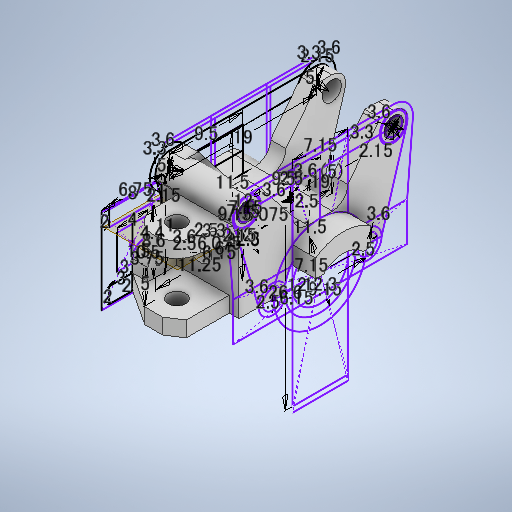
# Autodesk Inventor part: ikafly6.0_2.5d
Saved by Autodesk Inventor 2025 (Build 290162000, 162)
## iProperties
Created: 2024-06-20
Part Number: ikafly6.0_2.5d
Material: 一般
Document SubType Name: Modeling
Designer: Saigusa
Density: 1 g/cm^3
Appearance: 既定
Author: Saigusa
Autodesk Inventor part; units mm, degrees
ref_plane "YZ Plane" through (0, 0, 0) normal (1, 0, 0) x (0, 1, 0)
ref_plane "XZ Plane" through (0, 0, 0) normal (0, 1, 0) x (-1, 0, 0)
ref_plane "XY Plane" through (0, 0, 0) normal (0, 0, 1) x (1, 0, 0)
sketch "スケッチ1" plane through (0, 0, 0) normal (1, 0, 0) x (0, 1, 0)
  circle A0 centre (0, 0) radius 4.575
  circle A1 centre (0, 0) radius 3.575
  line L0 (0, 0) -> (0, 6)
  line L1 (0, 6) -> (0, -6)
  line L2 (0, 0) -> (11.5, 0)
  line L3 (11.5, 0) -> (11.5, 9.5)
  line L4 (11.5, 9.5) -> (11.5, -9.5)
  circle A2 centre (11.5, 9.5) radius 1.65
  circle A3 centre (11.5, -9.5) radius 1.65
  line L5 (0, 0) -> (0, 11.25)
  line L6 (0, 11.25) -> (0, -11.25)
  line L7 (-2.5, -11.25) -> (2.5, -11.25)
  line L8 (2.5, -11.25) -> (2.5, 11.25)
  line L9 (2.5, 11.25) -> (-2.5, 11.25)
  line L10 (-2.5, 11.25) -> (-2.5, -11.25)
  line L11 (-2.5, -11.25) -> (2.5, 11.25) construction
  line L12 (2.5, -11.25) -> (-2.5, 11.25) construction
  circle A4 centre (11.5, 9.5) radius 2.5
  circle A5 centre (11.5, -9.5) radius 2.5
  line L13 (2.5, 11.25) -> (11.2899, 11.9912)
  line L14 (2.5, -11.25) -> (11.2899, -11.9912)
  line L15 (14, 9.5) -> (14, -9.5)
  line L16 (0, -3.575) -> (14, -3.575)
  line L17 (0, 3.575) -> (14, 3.575)
  circle A6 centre (0, 0) radius 6
  line L18 (0, 0) -> (0, 6.15)
  line L19 (0, 6.15) -> (0, -6.15)
  circle A7 centre (0, 6.15) radius 1.25
  circle A8 centre (0, -6.15) radius 1.25
  line L20 (0, 0) -> (0, -6.075)
  line L21 (0, 0) -> (0, 6.075)
  circle A9 centre (0, -6.075) radius 1.25
  circle A10 centre (0, 6.075) radius 1.25
  circle A11 centre (11.5, 9.5) radius 1.075
  circle A12 centre (11.5, -9.5) radius 1.075
  circle A13 centre (11.5, -9.5) radius 1.8
  circle A14 centre (11.5, 9.5) radius 1.8
  line L22 (11.5, -9.5) -> (13.3, -9.5)
  line L23 (11.5, 9.5) -> (13.3, 9.5)
  line L24 (13.3, -9.5) -> (13.3, 9.5)
  circle A15 centre (0, -6.15) radius 1.8
  circle A16 centre (0, 6.15) radius 1.8
  line L25 (0, -7.95) -> (10.9858, -11.225)
  line L26 (0, 7.95) -> (10.9858, 11.225)
  line L27 (0, 11.3) -> (0, 0)
  line L28 (0, 0) -> (11.5, 0)
  line L29 (11.5, 0) -> (11.5, 11.3)
  line L30 (0, 0) -> (8.6, 0)
  line L31 (8.6, 0) -> (8.6, 10.5138)
  line L32 (8.6, 10.5138) -> (0, 10.5138)
  line L33 (0, 10.5138) -> (0, 0)
  line L34 (0, 10.5138) -> (2, 10.5138)
  line L35 (2, 10.5138) -> (2, 14.2638)
  line L36 (2, 14.2638) -> (0, 14.2638)
  line L37 (0, 14.2638) -> (0, 10.5138)
  line L38 (0, 14.2638) -> (2, 14.2638)
  line L39 (2, 14.2638) -> (2, 17.2638)
  line L40 (2, 17.2638) -> (0, 17.2638)
  line L41 (0, 17.2638) -> (0, 14.2638)
  line L42 (0, 10.5138) -> (8.6, 10.5138)
  line L43 (8.6, 10.5138) -> (8.6, 14.2638)
  line L44 (8.6, 14.2638) -> (0, 14.2638)
  line L45 (0, 14.2638) -> (0, 10.5138)
  line L46 (8.6, 10.5138) -> (10.6, 10.5138)
  line L47 (10.6, 10.5138) -> (10.6, 17.2638)
  line L48 (10.6, 17.2638) -> (8.6, 17.2638)
  line L49 (8.6, 17.2638) -> (8.6, 10.5138)
  line L50 (3.1, 16.2638) -> (7.5, 16.2638)
  line L51 (7.5, 16.2638) -> (7.5, 12.2638)
  line L52 (7.5, 12.2638) -> (3.1, 12.2638)
  line L53 (3.1, 12.2638) -> (3.1, 16.2638)
  line L54 (3.1, 16.2638) -> (7.5, 12.2638) construction
  line L55 (7.5, 16.2638) -> (3.1, 12.2638) construction
  line L56 (3.1, 14.2638) -> (3.6, 14.2638)
  line L57 (3.6, 14.2638) -> (3.6, 12.7638)
  line L58 (3.6, 12.7638) -> (3.1, 12.7638)
  line L59 (3.1, 12.7638) -> (3.1, 14.2638)
  circle A17 centre (3.6, 12.7638) radius 0.5
  circle A18 centre (3.6, 12.7638) radius 1.5
  line L60 (3.6, 12.7638) -> (5.1, 12.7638)
  line L61 (5.1, 12.7638) -> (5.1, 10.5138)
  line L62 (5.1, 10.5138) -> (3.6, 10.5138)
  line L63 (3.6, 10.5138) -> (3.6, 12.7638)
  line L64 (11.5, 7.7) -> (0, 7.7)
  line L65 (10.6, 10.5138) -> (11.1423, 10.5138)
  line L66 (0, 7.7) -> (10.6, 7.7)
  line L67 (10.6, 7.7) -> (10.6, 10.5138)
  line L68 (10.6, 10.5138) -> (0, 10.5138)
  line L69 (0, 10.5138) -> (0, 7.7)
  line L70 (-0.2, 18.2638) -> (10.8, 18.2638)
  line L71 (10.8, 18.2638) -> (10.8, 10.2638)
  line L72 (10.8, 10.2638) -> (-0.2, 10.2638)
  line L73 (-0.2, 10.2638) -> (-0.2, 18.2638)
  line L74 (-0.2, 18.2638) -> (10.8, 10.2638) construction
  line L75 (10.8, 18.2638) -> (-0.2, 10.2638) construction
  point P0 (0, 4.575)
  point P1 (0, -4.575)
  point P2 (2.5, 3.575)
  point P3 (2.5, 2.5555)
  point P4 (2.5, -2.5555)
  point P5 (2.5, -3.575)
  point P6 (0, 7.4)
  point P7 (0, 4.9)
  point P8 (0, -4.9)
  point P9 (0, -7.4)
  point P10 (2.5, 5.4544)
  point P11 (2.5, -5.4544)
  point P12 (4.8186, 3.575)
  point P13 (4.8186, -3.575)
  point P14 (2.8548, 3.575)
  point P15 (2.8548, -3.575)
  point P16 (0, 7.95)
  point P17 (2.5, -8.6953)
  point P18 (2.5, 8.6953)
  point P19 (5.3, 14.2638)
  point P20 (3.2258, 11.3112)
  point P21 (3.6, 11.3428)
  point P22 (3.6, 11.2638)
  point P23 (11.5, 7.85)
  point P24 (10.1982, 10.5138)
  point P25 (10.6, 8.1171)
  point P26 (11.5, 8.425)
  point P27 (11.5, 10.575)
  point P28 (10.0126, 10.5138)
  point P29 (10.6, 11.933)
  point P30 (8.6, 11.7643)
  point P31 (10.7435, 10.2638)
  point P32 (10.8, 10.3159)
  point P33 (10.8, 11.1696)
  point P34 (10.6, 11.11)
  point P35 (8.6, 10.2638)
  point P36 (10.8, 10.5138)
  dimension "d110" = 2.15
  dimension "d114" = 3.6
  dimension "d115" = 3.6
  dimension "d0" = 9.15
  dimension "d1" = 7.15
  dimension "d2" = 6
  dimension "d3" = 12
  dimension "d6" = 11.5
  dimension "d7" = 9.5
  dimension "d8" = 19
  dimension "d9" = 3.3
  dimension "d10" = 3.3
  dimension "d11" = 11.25
  dimension "d12" = 22.5
  dimension "d13" = 5
  dimension "d14" = 5
  dimension "d15" = 5
  dimension "d28" = 12
  dimension "d29" = 6.15
  dimension "d30" = 12.3
  dimension "d31" = 2.5
  dimension "d32" = 2.5
  dimension "d99" = 6.075
  dimension "d100" = 6.075
  dimension "d101" = 2.5
  dimension "d102" = 2.5
  dimension "d111" = 2.15
  dimension "d112" = 3.6
  dimension "d113" = 3.6
  dimension "d133" = 8.6
  dimension "d134" = 2
  dimension "d135" = 3.75
  dimension "d136" = 2
  dimension "d137" = 3
  dimension "d138" = 2
  dimension "d139" = 6.75
  dimension "d140" = 4.4
  dimension "d141" = 4
  dimension "d142" = 0.5
  dimension "d143" = 1.5
  dimension "d144" = 3
  dimension "d174" = 11
  dimension "d175" = 8
  constraints: 152 end point, 25 parallel, 19 coincident, 18 point on line, 15 centre point, 15 perpendicular, 13 horizontal, 12 point on circle, 8 tangent, 7 midpoint, 2 vertical alignment, 1 horizontal alignment, 1 vertical, 9 other
  measures "d0" diameter of A0
  measures "d1" diameter of A1
  measures "d2" distance of L0.start L0.end
  measures "d3" distance of L0.end L1.end
  measures "d6" distance of L0.start L2.end
  measures "d7" distance of L2.end L3.end
  measures "d8" distance of L3.end L4.end
  measures "d9" diameter of A2
  measures "d10" diameter of A3
  measures "d11" distance of L0.start L5.end
  measures "d12" distance of L5.end L6.end
  measures "d13" distance of L9.end L8.end
  measures "d14" diameter of A4
  measures "d15" diameter of A5
  measures "d28" diameter of A6
  measures "d29" distance of L18.start L18.end
  measures "d30" distance of L18.end L19.end
  measures "d31" diameter of A7
  measures "d32" diameter of A8
  measures "d99" distance of L18.start L20.end
  measures "d100" distance of L18.start L21.end
  measures "d101" diameter of A9
  measures "d102" diameter of A10
  measures "d111" diameter of A12
  measures "d112" diameter of A13
  measures "d113" diameter of A14
  measures "d133" distance of L32.end L31.end
  measures "d134" distance of L36.end L35.end
  measures "d135" distance of L35.end L34.end
  measures "d136" distance of L40.end L39.end
  measures "d137" distance of L39.end L38.end
  measures "d138" distance of L48.end L47.end
  measures "d139" distance of L47.end L46.end
  measures "d140" distance of L51.end L52.end
  measures "d141" distance of L50.end L51.end
  measures "d142" distance of L57.end L58.end
  measures "d143" distance of L56.end L57.end
  measures "d144" diameter of A18
  measures "d174" distance of L71.end L72.end
  measures "d175" distance of L70.end L71.end
extrude "押し出し7" add sketch "スケッチ1" along normal blind 2 contours L2 A6 L16 A0 | A0 L17 A6 L2 | A0 L8 A6 L17 | L16 A6 L8 A0 | A6 L17 L31 L2 | L2 L4 L16 A6 | A0 A16 A6 L8 | A6 L8 L64 L31 L17 | L8 A6 A15 A0 | L16 L4 A5 L25 L8 A6 | L31 L17 L3 L2 | A0 L0 A10 A6 A16 | A6 A16 L64 L8 | L31 L64 A4 L3 L17 | A15 A6 A9 L1 A0 | L8 L25 A15 A6 | L16 L24 A5 L4 | L4 L3 L17 L24 L16 | A6 A10 L5 L64 A16 | L64 A16 L26 L8 | L8 L26 L72 L31 L64 | L3 A4 L24 L17 | L31 L72 A4 L64 | A15 L6 A8 A6 | A5 L24 A13 L4 | L4 A13 L25 A5 | L0 A7 A6 A10 | L64 L5 A16 | A4 L64 L3 | L3 A14 L24 A4 | L72 L26 L31 | L31 L46 A4 L72 | A4 L72 A14 L67 L64 | A9 A6 A8 L1 | A13 L22 A3 L4 | L4 A3 L22 A13 | A14 L67 A2 L3 | L3 A2 L23 A14 | L64 L67 A14 | L26 A4 L46 | A4 L46 A14 L72 | L23 A2 L29 A14 | A14 L72 A2 L67 | L26 L47 A14 L46 A4 | A14 L46 A2 L72 | L29 A2 L71 A14 | L26 L71 A14 L47 | A14 L47 A2 L46 | A14 L71 L26 | A14 L71 A2 L47 picked at (1.3383, 5.2331) picked at (1.3383, -5.2331) picked at (0.0969, 4.8614) picked at (0.0969, -4.8614)
extrude "押し出し8" add sketch "スケッチ1" along normal blind 10 contours L2 A6 L16 A0 | A0 L17 A6 L2 | A0 L8 A6 L17 | L16 A6 L8 A0 | A6 L17 L31 L2 | L2 L4 L16 A6 | A0 A16 A6 L8 | L8 A6 A15 A0 | L31 L17 L3 L2 | A0 L0 A10 A6 A16 | A6 A16 L64 L8 | A15 A6 A9 L1 A0 | L8 L25 A15 A6 | L4 L3 L17 L24 L16 | A6 A10 L5 L64 A16 | L64 A16 L26 L8 | A15 L6 A8 A6 | L24 L17 L15 L16 | L0 A7 A6 A10 | A6 L5 A10 | L64 L5 A16 | A9 A6 A8 L1 | L0 A6 A7 | A8 A6 L1 | A8 L6 A6 picked at (1.3383, 5.2331) picked at (1.3383, -5.2331) picked at (0.0969, 4.8614) picked at (0.0969, -4.8614) picked at (0.2292, 5.6392) picked at (0.2292, -5.6392)
sketch "スケッチ6" plane through (10, 0, 0) normal (1, 0, 0) x (0, 0, -1)
  line L0 (0, 0) -> (-6.15, 0)
  line L1 (-6.15, 0) -> (6.15, 0)
  circle A0 centre (-6.15, 0) radius 1.25
  circle A1 centre (6.15, 0) radius 1.25
  line L2 (-11.25, 2.5) -> (11.25, 2.5)
  line L3 (11.25, 2.5) -> (11.25, -2.5)
  line L4 (11.25, -2.5) -> (-11.25, -2.5)
  line L5 (-11.25, -2.5) -> (-11.25, 2.5)
  line L6 (-11.25, 2.5) -> (11.25, -2.5) construction
  line L7 (11.25, 2.5) -> (-11.25, -2.5) construction
  line L8 (0, 0) -> (0, 11.5)
  line L9 (0, 11.5) -> (-9.5, 11.5)
  line L10 (-9.5, 11.5) -> (9.5, 11.5)
  circle A2 centre (-9.5, 11.5) radius 1.65
  circle A3 centre (9.5, 11.5) radius 1.65
  circle A4 centre (0, 0) radius 6
  circle A5 centre (0, 0) radius 4.575
  arc A6 (11.9912, 11.2899) -> (9.5, 14) centre (9.5, 11.5) ccw
  line L11 (11.25, 2.5) -> (11.9912, 11.2899)
  line L12 (-11.25, 2.5) -> (-11.9912, 11.2899)
  line L13 (-9.5, 14) -> (9.5, 14)
  circle A7 centre (0, 0) radius 3.575
  line L14 (-3.575, 14) -> (-3.575, 4.8186)
  line L15 (3.575, -14) -> (-3.575, -14)
  line L16 (-3.575, 14) -> (3.575, 14)
  line L17 (3.575, 14) -> (3.575, -14)
  line L18 (3.575, -14) -> (-3.575, 14) construction
  line L19 (-3.575, -14) -> (3.575, 14) construction
  circle A8 centre (-9.5, 11.5) radius 1.075
  circle A9 centre (9.5, 11.5) radius 1.075
  circle A10 centre (9.5, 11.5) radius 1.8
  circle A11 centre (-9.5, 11.5) radius 1.8
  line L20 (-9.5, 11.5) -> (-9.5, 13.3)
  line L21 (-9.5, 13.3) -> (9.5, 13.3)
  circle A12 centre (-6.15, 0) radius 1.8
  circle A13 centre (6.15, 0) radius 1.8
  line L22 (-7.95, 0) -> (-11.225, 10.9858)
  line L23 (4.575, 0) -> (7.95, 0)
  line L24 (7.95, 0) -> (11.225, 10.9858)
  line L25 (3.575, -13.3) -> (-3.575, -13.3)
  line L26 (-3.575, -13.3) -> (-3.575, 13.3)
  line L27 (-3.575, 13.3) -> (3.575, 13.3)
  line L28 (3.575, 13.3) -> (3.575, -13.3)
  line L29 (3.575, -13.3) -> (-3.575, 13.3) construction
  line L30 (-3.575, -13.3) -> (3.575, 13.3) construction
  point P0 (-5.4544, 2.5)
  point P1 (5.4544, 2.5)
  point P2 (-3.575, 11.5)
  point P3 (-2.5555, 2.5)
  point P4 (2.5555, 2.5)
  point P5 (3.575, 2.5)
  point P6 (3.575, 11.5)
  point P7 (-8.6953, 2.5)
  point P8 (8.6953, 2.5)
  point P9 (3.575, 0)
  point P10 (-3.575, 11.5)
  point P11 (3.575, -2.5)
  point P12 (0, 2.5)
  point P13 (0, 3.575)
  point P14 (3.575, 4.8186)
  point P15 (-3.575, 4.8186)
  point P16 (-3.575, 2.5)
  dimension "d69" = 12
  dimension "d120" = 3.6
  dimension "d121" = 3.6
  dimension "d56" = 6.15
  dimension "d57" = 12.3
  dimension "d58" = 2.5
  dimension "d59" = 2.5
  dimension "d62" = 11.5
  dimension "d63" = 9.5
  dimension "d64" = 19
  dimension "d65" = 3.3
  dimension "d67" = 3.3
  dimension "d70" = 9.15
  dimension "d79" = 7.15
  dimension "d116" = 2.15
  dimension "d117" = 2.15
  dimension "d118" = 3.6
  dimension "d119" = 3.6
  dimension "d124" = 7.15
  dimension "d125" = 26.6
  constraints: 62 end point, 13 coincident, 11 centre point, 6 midpoint, 6 point on circle, 5 horizontal, 5 parallel, 4 tangent, 3 perpendicular, 2 horizontal alignment, 2 point on line, 2 vertical, 5 other
  measures "d56" distance of L0.start L0.end
  measures "d57" distance of L0.end L1.end
  measures "d58" diameter of A0
  measures "d59" diameter of A1
  measures "d62" distance of L0.start L8.end
  measures "d63" distance of L8.end L9.end
  measures "d64" distance of L9.end L10.end
  measures "d65" diameter of A2
  measures "d67" diameter of A3
  measures "d70" diameter of A5
  measures "d79" diameter of A7
  measures "d116" diameter of A8
  measures "d117" diameter of A9
  measures "d118" diameter of A10
  measures "d119" diameter of A11
  measures "d124" distance of L26.end L27.end
  measures "d125" distance of L25.end L26.end
extrude "押し出し9" add sketch "スケッチ6" against normal blind 2 contours L2 L22 A11 L9 L14 A4 | L14 L9 L8 A4 | A4 L17 L10 A10 L24 L2 | A4 L8 L10 L17 | L14 L21 L17 L10 L9 | L9 A11 L21 L14 | L17 L21 A10 L10 | A11 L20 A2 L9 | L9 A2 L20 A11 | A10 | A2 L20 A8 L9 | L9 A8 L20 A2 | A3
extrude "押し出し10" add sketch "スケッチ1" against normal blind 0.5 contours L2 A6 L16 A0 | A0 L17 A6 L2 | A6 L17 L31 L2 | L2 L4 L16 A6 | L31 L17 L3 L2 | L4 L3 L17 L24 L16 | L24 L17 L15 L16
sketch "スケッチ7" plane through (-0.5, 0, 0) normal (-1, 0, 0) x (0, 0, 1)
  circle A0 centre (0, 0) radius 3.575
  line L0 (-9.5, 14) -> (9.5, 14)
  line L1 (-3.575, 14) -> (3.575, 14)
  circle A1 centre (0, 0) radius 4.575
  line L2 (-11.25, 0) -> (-11.25, 2.5)
  line L3 (11.25, -2.5) -> (-11.25, -2.5)
  line L4 (-11.25, -2.5) -> (-11.25, 2.5)
  line L5 (-11.25, 2.5) -> (11.25, 2.5)
  line L6 (11.25, 2.5) -> (11.25, -2.5)
  line L7 (11.25, -2.5) -> (-11.25, 2.5) construction
  line L8 (-11.25, -2.5) -> (11.25, 2.5) construction
  line L9 (-3.575, 14) -> (-3.575, 0)
  line L10 (3.575, 14) -> (3.575, 0)
  point P0 (-3.575, 2.5)
  point P1 (-2.5555, 2.5)
  point P2 (2.5555, 2.5)
  point P3 (3.575, 2.5)
  dimension "d75" = 7.15
  dimension "d76" = 5
  constraints: 22 end point, 2 centre point, 2 coincident, 2 midpoint, 2 parallel, 2 point on circle, 2 point on line, 2 tangent, 1 horizontal, 1 perpendicular
  measures "d75" diameter of A0
  measures "d76" distance of L3.end L2.end
extrude "押し出し11" add sketch "スケッチ7" along normal blind 3 contours A0 L5 L9 A1 L10 | A1 L9 L0 L10
extrude "押し出し12" add sketch "スケッチ6" along normal blind 3 contours L2 L26 A5 L8 A7 | A7 L8 A5 L17 L2 | L26 A4 L8 A5 | A5 L8 A4 L17
sketch "スケッチ8" plane through (13, 0, 0) normal (1, 0, 0) x (0, 0, -1)
  line L0 (-3.575, 2.5) -> (-3.575, 14) projected
  line L1 (3.575, 14) -> (3.575, 2.5) projected
  line L2 (-3.575, 14) -> (3.575, 14)
  line L3 (3.575, 14) -> (3.575, 2.5)
  line L4 (3.575, 2.5) -> (-3.575, 2.5)
  line L5 (-3.575, 2.5) -> (-3.575, 14)
  circle A0 centre (0, 0) radius 6
  line L6 (-3.575, 14) -> (3.575, 14)
  line L7 (3.575, 14) -> (3.575, 6)
  line L8 (3.575, 6) -> (-3.575, 6)
  line L9 (-3.575, 6) -> (-3.575, 14)
  dimension "d89" = 12
  constraints: 16 end point, 4 parallel, 2 horizontal, 2 perpendicular, 1 centre point, 1 coincident, 1 point on line
  measures "d89" diameter of A0
extrude "押し出し13" cut sketch "スケッチ8" against normal blind 16.5 contours L0 L2 L1 L8
fillet "フィレット1" radius 2 8 edges at (9, 6, 3.575) (9, 6, -3.575) (1, 6, -3.575) (5, 6, 3.575) (5, 6, -3.575) (1, 6, 3.575) (-1.75, 6, 3.575) (-1.75, 6, -3.575)
sketch "スケッチ9" plane through (10, 0, 0) normal (1, 0, 0) x (0, 0, -1)
  arc A0 (2.5555, 2.5) -> (-2.5555, 2.5) centre (0, 0) ccw projected
  line L0 (0, 0) -> (0, 11.5)
  line L1 (0, 11.5) -> (-9.5, 11.5)
  circle A1 centre (9.5, 11.5) radius 1.65 projected
  line L2 (-9.5, 11.5) -> (9.5, 11.5)
  circle A2 centre (-9.5, 11.5) radius 2.5
  circle A3 centre (9.5, 11.5) radius 2.5
  arc A4 (-3.575, 8) -> (-1.575, 6) centre (-1.575, 8) ccw
  line L3 (-3.575, 8) -> (-7.5334, 13.0435)
  arc A5 (1.575, 6) -> (3.575, 8) centre (1.575, 8) ccw
  line L4 (3.575, 8) -> (7.5334, 13.0435)
  line L5 (9.5, 14) -> (3.575, 14)
  line L6 (-3.575, 8) -> (3.575, 8)
  line L7 (3.575, 8) -> (3.575, 14)
  line L8 (3.575, 14) -> (-3.575, 14)
  line L9 (-3.575, 14) -> (-3.575, 8)
  line L10 (-3.575, 8) -> (-9.5, 8)
  line L11 (-9.5, 8) -> (-9.5, 14)
  line L12 (-9.5, 14) -> (-3.575, 14)
  line L13 (-3.575, 14) -> (-3.575, 8)
  line L14 (3.575, 8) -> (9.5, 8)
  line L15 (9.5, 8) -> (9.5, 14)
  line L16 (9.5, 14) -> (3.575, 14)
  line L17 (3.575, 14) -> (3.575, 8)
  dimension "d93" = 11.5
  dimension "d94" = 9.5
  dimension "d95" = 5
  dimension "d96" = 5
  constraints: 36 end point, 7 point on circle, 6 parallel, 4 centre point, 4 perpendicular, 3 horizontal, 2 coincident, 2 tangent, 1 vertical
  measures "d93" distance of L0.start L0.end
  measures "d94" distance of L0.end L1.end
  measures "d95" diameter of A2
  measures "d96" diameter of A3
extrude "押し出し14" cut sketch "スケッチ9" against normal blind 16.5 contours L3 L1 L9 | L7 L2 L4 | L1 L3 A2 L12 L9 | L7 L5 A3 L4 L2
hole "穴2" at (0, 0, 6.075) at (0, 0, -6.075) direction (1, 0, 0) diameter 2.45 depth 2
extrude "押し出し15" add sketch "スケッチ1" along normal blind 2 contours A3 L22 A12 L4 | L4 A12 L22 A3 | A2 L67 A11 L3 | L3 A11 L23 A2 | A2 L72 L67 A11 | L23 A11 L29 A2 | A2 L46 L67 L72 | L29 A11 L65 L71 A2 | A2 L47 L46 | L72 A11 L67 | L67 L65 L71 A11 L72 | L71 L65 L47 A2 | A11 L71 L65
extrude "押し出し16" add sketch "スケッチ1" along normal blind 10 contours L64 A16 L26 L8 | L8 L26 L72 L31 L64 | L31 L72 A4 L64 | L26 L5 L72 L8 | L8 L72 L26 | L64 L5 A16 | L72 L26 L31 | L31 L46 A4 L72 | A4 L72 A14 L67 L64 | L72 L5 L32 L8 | L8 L32 L26 L72 | A14 L67 A2 L3 | L3 A2 L23 A14 | L64 L67 A14 | A4 L46 A14 L72 | A2 L67 A11 L3 | L3 A11 L23 A2 | L23 A2 L29 A14 | A14 L72 A2 L67 | A14 L46 A2 L72 | A2 L72 L67 A11 | L23 A11 L29 A2 | L29 A2 L71 A14 | A14 L47 A2 L46 | A2 L46 L67 L72 | L29 A11 L65 L71 A2 | A14 L71 A2 L47 | A2 L47 L46 | L72 A11 L67 | L67 L65 L71 A11 L72 | L71 L65 L47 A2 | A11 L71 L65
extrude "押し出し17" add sketch "スケッチ1" along normal blind 2 contours L32 L35 L9 L8 | L8 L13 A18 L63 L32 | L32 L63 A18 L13 L61 | L9 L35 L44 L53 A18 L13 | L32 L5 L9 L35 | L13 A18 L52 L61 | L9 L27 L37 L36 L35 | A18 L53 L52 L63 L13 | L13 L63 A18 | L63 L13 A18 | L13 L63 L52 A18 | L52 A18 L61 | A18 L57 A17 L53 | L53 L44 A18 | L52 A17 L60 A18 | L60 A17 L57 A18 | L52 L53 A17
sketch "スケッチ11" plane through (0, 0, 4.575) normal (0, -1, 0) x (1, 0, 0)
  line L0 (0, 9.6888) -> (0, 2.725) projected
  line L1 (0, 9.6888) -> (2, 9.6888)
  line L2 (2, 9.6888) -> (2, 5.9388)
  line L3 (2, 5.9388) -> (0, 5.9388)
  line L4 (0, 5.9388) -> (0, 9.6888)
  line L5 (2, 9.6888) -> (5.75, 9.6888)
  line L6 (2, 9.6888) -> (5.75, 9.6888) construction
  circle A0 centre (5.75, 9.6888) radius 1.15
  line L7 (5.75, 9.6888) -> (4.6, 9.6888)
  line L8 (4.6, 9.6888) -> (4.6, 12.6888)
  line L9 (4.6, 12.6888) -> (5.75, 12.6888)
  line L10 (5.75, 12.6888) -> (5.75, 9.6888)
  line L11 (0, 9.6888) -> (4.6, 12.6888)
  line L12 (2, 5.9388) -> (8.75, 5.9388)
  line L13 (8.75, 5.9388) -> (8.75, 12.6888)
  line L14 (8.75, 12.6888) -> (2, 12.6888)
  line L15 (2, 12.6888) -> (2, 5.9388)
  line L16 (5.75, 9.6888) -> (6.9, 9.6888)
  line L17 (6.9, 9.6888) -> (6.9, 12.6888)
  line L18 (6.9, 12.6888) -> (5.75, 12.6888)
  line L19 (5.75, 12.6888) -> (5.75, 9.6888)
  line L20 (6.9, 9.6888) -> (11.5, 9.6888)
  line L21 (6.9, 9.6888) -> (11.5, 9.6888) construction
  line L22 (11.5, 9.6888) -> (6.9, 12.6888)
  point P0 (0, -4.575)
  point P1 (8.75, 11.4822)
  dimension "d157" = 2
  dimension "d158" = 3.75
  dimension "d159" = 3.75
  dimension "d160" = 0
  dimension "d161" = 2.3
  dimension "d162" = 3
  dimension "d163" = 6.75
  dimension "d164" = 4.6
  dimension "d165" = 0
  constraints: 44 end point, 8 horizontal, 8 parallel, 4 perpendicular, 2 collinear, 1 centre point, 1 coincident, 1 point on line
  measures "d157" distance of L2.end L3.end
  measures "d158" distance of L1.end L2.end
  measures "d159" distance of L1.end L5.end
  measures "d160" distance between parallel lines of L5 L6
  measures "d161" diameter of A0
  measures "d162" distance of L7.end L8.end
  measures "d163" distance of L14.end L13.end
  measures "d164" distance of L16.end L20.end
  measures "d165" distance between parallel lines of L20 L21
extrude "押し出し19" add sketch "スケッチ11" against normal blind 2 contours L11 L15 L1 | L5 A0 L20 L13 L12 L2 | L15 L11 L8 L5 | L8 L9 L10 A0 | A0 L10 L14 L17 | L17 L22 L13 L20
ref_plane "作業平面2" through (0, 8.6, 4.575) normal (0, 1, 0) x (1, 0, 0)
sketch "スケッチ13" plane through (0, 8.6, 4.575) normal (0, 1, 0) x (1, 0, 0)
  circle A0 centre (5.75, -9.6888) radius 1.15 projected
  circle A1 centre (5.75, -9.6888) radius 1.15
  circle A2 centre (5.75, -9.6888) radius 3
  line L0 (8.75, -11.4822) -> (8.75, -5.9388) projected
  line L1 (5.75, -9.6888) -> (8.75, -9.6888)
  line L2 (8.75, -9.6888) -> (8.75, -5.9388)
  line L3 (8.75, -5.9388) -> (5.75, -5.9388)
  line L4 (5.75, -5.9388) -> (5.75, -9.6888)
  line L5 (5.75, -9.6888) -> (2.75, -9.6888)
  line L6 (2.75, -9.6888) -> (2.75, -5.9388)
  line L7 (2.75, -5.9388) -> (5.75, -5.9388)
  line L8 (5.75, -5.9388) -> (5.75, -9.6888)
  line L9 (8, -5.9388) -> (10, -5.9388) projected
  line L10 (8.75, -5.9388) -> (10, -5.9388)
  line L11 (10, -5.9388) -> (8.75, -9.6888)
  point P0 (0, 4.575)
  dimension "d169" = 6
  constraints: 20 end point, 4 parallel, 3 horizontal, 2 coincident, 2 perpendicular, 2 point on line, 1 centre point, 3 other
extrude "押し出し20" add sketch "スケッチ13" along normal blind 2 contours L1 A2 L5 A0 | A0 L4 A2 L1 | A0 L5 A2 L4 | A2 L4 L3 L0 | L0 L9 L11 | A2 L6 L7 L4
hole "穴3" at (10, 11.5, 9.5) at (10, 11.5, -9.5) direction (-1, 0, 0) diameter 2.5 end through all
extrude "押し出し21" cut sketch "スケッチ1" along normal up to surface (2.75 mm away) contours L43 L13 L47 A4 L26 | L26 A4 L46 | L26 L47 A14 L46 A4 | A4 L47 L26 | L26 L71 A14 L47 | A14 L47 A2 L46 | A14 L71 A2 L47 | A2 L47 L46 | L71 L65 L47 A2
sketch "スケッチ14" plane through (0, 5.1, 10.5138) normal (0, 0, 1) x (1, 0, 0)
  line L0 (0, 0.9) -> (0, -1.1) projected
  line L1 (0, -0.0005) -> (0, 5.9995)
  line L2 (0, 0) -> (2, 0) projected
  line L3 (0, 0) -> (5, 0)
  line L4 (5, 0) -> (5, 0.2)
  line L5 (5, 0.2) -> (0, 0.2)
  line L6 (0, 0.2) -> (0, 0)
  point P0 (0, -5.1)
  dimension "d176" = 6
  dimension "d177" = 5
  dimension "d178" = 0.2
  constraints: 10 end point, 2 parallel, 1 collinear, 1 horizontal, 1 perpendicular, 1 point on line
  measures "d176" distance of L1.start L1.end
  measures "d177" distance of L5.end L4.end
  measures "d178" distance of L4.end L3.end
hole "穴4" at (5, 5.3, 10.5138) direction (0, 0, -1) diameter 3 depth 3
